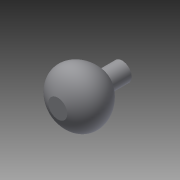
# Autodesk Inventor part: pounder
Saved by Autodesk Inventor 2015 (Build 190159000, 159)
## iProperties
Created: 2014-07-11
Part Number: pounder
Material: Generic
Document SubType Name: Modeling
Designer: shohei
Density: 1 g/cm^3
Appearance: Default
Author: shohei
Autodesk Inventor part; units mm, degrees
ref_plane "YZ Plane" through (0, 0, 0) normal (1, 0, 0) x (0, 1, 0)
ref_plane "XZ Plane" through (0, 0, 0) normal (0, 1, 0) x (-1, 0, 0)
ref_plane "XY Plane" through (0, 0, 0) normal (0, 0, 1) x (1, 0, 0)
sketch "Sketch1" plane through (0, 0, 0) normal (0, 0, 1) x (1, 0, 0)
  spline S0 degree 3 poles (-5, 0) (-19.6099, 5.4165) (-15.2363, 18.1555) (-5, 24) knots 0 0 0 0 1 1 1 1
  line L0 (-5, 24) -> (-5, 34)
  line L1 (-5, 34) -> (0, 34)
  line L2 (0, -7.0933) -> (0, 40.8489) projected
  line L3 (-5, 0) -> (0, 0)
  line L4 (0, 34) -> (0, 0)
  line L5 (-18.5589, 0) -> (3.0931, 0) projected
  point P0 (-14, 8)
  point P1 (-13, 16)
  dimension "d0" = 5
  dimension "d1" = 5
  dimension "d7" = 14
  dimension "d8" = 13
  dimension "d9" = 8
  dimension "d10" = 8
  dimension "d11" = 8
  dimension "d12" = 10
  constraints: 8 end point, 2 perpendicular, 1 horizontal, 1 vertical, 5 other
  measures "d0" distance between parallel lines of L2 L0
  measures "d1" distance from line of L2 point (-5, 0)
  measures "d7" distance from line of L2 point (-14, 8)
  measures "d8" distance from line of L2 point (-13, 16)
  measures "d9" distance from line of L5 point (-14, 8)
  measures "d10" vertical distance of point (-14, 8) point (-13, 16)
  measures "d11" horizontal distance of L0.start point (-13, 16)
  measures "d12" distance from line of L0.start L1
revolve "Revolution1" add sketch "Sketch1" angle 360 about axis through (0, -10, 0) along (0, 1, 0)
sketch "Sketch3" plane through (0, 34, 0) normal (0, 1, 0) x (1, 0, 0)
  circle A0 centre (0, 0) radius 1.5
  dimension "d4" = 3
  constraints: 1 centre point, 1 coincident
  measures "d4" diameter of A0
extrude "Extrusion1" cut sketch "Sketch3" against normal blind 5
body "Solid1"
